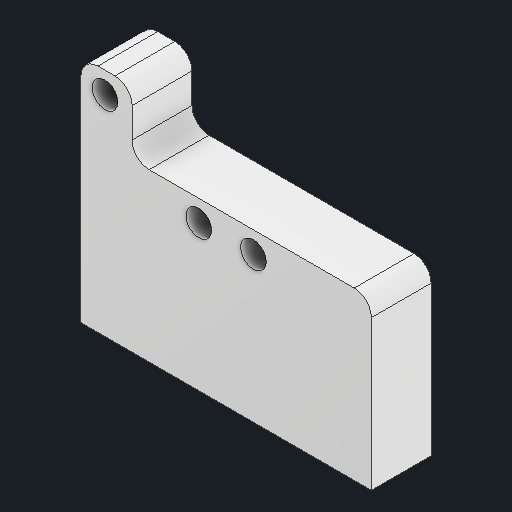
# Autodesk Inventor part: Pixy2Mount
Saved by Autodesk Inventor 2025 (Build 290162000, 162)
## iProperties
Created: 2024-05-22
Part Number: Pixy2Mount
Material: PC/ABS Plastic
Document SubType Name: Modeling
Designer: avsar
Density: 1.1 g/cm^3
Appearance: Smooth - White
Author: avsar
Autodesk Inventor part; units mm, degrees
ref_plane "YZ Plane" through (0, 0, 0) normal (1, 0, 0) x (0, 1, 0)
ref_plane "XZ Plane" through (0, 0, 0) normal (0, 1, 0) x (-1, 0, 0)
ref_plane "XY Plane" through (0, 0, 0) normal (0, 0, 1) x (1, 0, 0)
sketch "Sketch1" plane through (0, 0, 0) normal (0, 1, 0) x (-1, 0, 0)
  circle A0 centre (0, 0) radius 2
  circle A1 centre (12, 0) radius 2
  line L0 (0, 0) -> (0, 2) construction
  circle A2 centre (-12, 0) radius 2
  line L1 (17, 3.5) -> (-17, 3.5)
  line L2 (-17, 3.5) -> (-17, -3.5)
  line L3 (-17, -3.5) -> (17, -3.5)
  line L4 (17, -3.5) -> (17, 3.5)
  line L5 (17, 3.5) -> (-17, -3.5) construction
  line L6 (-17, 3.5) -> (17, -3.5) construction
  dimension "d0" = 4
  dimension "d1" = 4
  dimension "d2" = 12
  dimension "d3" = 34
  dimension "d4" = 7
  constraints: 14 end point, 2 centre point, 2 midpoint, 2 parallel, 1 coincident, 1 horizontal, 1 horizontal alignment, 1 perpendicular, 1 symmetric about line, 1 vertical, 1 vertical alignment, 3 other
  measures "d1" diameter of A1
  measures "d2" distance of point (0, 0) A1.centre
  measures "d3" distance of L3.end L2.end
  measures "d4" distance of L2.end L1.end
extrude "Extrusion1" add sketch "Sketch1" along normal blind 27 contours A0 | A1 | A2 | L4 L3 L2 L1
extrude "Extrusion2" cut sketch "Sketch1" along normal blind 8 contours A0 | A1 | A2
sketch "Sketch2" plane through (-17, 0, 3.5) normal (0, 0, 1) x (1, 0, 0)
  circle A0 centre (20.2, 17) radius 1.5
  circle A1 centre (13.8, 17) radius 1.5
  circle A2 centre (2.825, 24.5) radius 1.5
  line L0 (13.8, 17) -> (20.2, 17) construction
  line L1 (0, 0) -> (34, 0) projected
  line L2 (0, 27) -> (34, 27) construction
  point P0 (17, 0)
  point P1 (17, 17)
  point P2 (17, 0)
  point P3 (17, 27)
  dimension "d9" = 3
  dimension "d10" = 3
  dimension "d11" = 3
  dimension "d12" = 6.4
  dimension "d13" = 10.975
  dimension "d14" = 7.5
  dimension "d15" = 10
  constraints: 3 centre point, 3 midpoint, 2 end point, 1 horizontal, 1 horizontal alignment, 1 vertical alignment
  measures "d9" diameter of A0
  measures "d10" diameter of A1
  measures "d11" diameter of A2
  measures "d12" distance of L0.end L0.start
  measures "d13" horizontal distance of L0.start A2.centre
  measures "d14" vertical distance of A2.centre L0.start
  measures "d15" distance of point (17, 27) point (17, 17)
extrude "Extrusion3" cut sketch "Sketch2" against normal through all
sketch "Sketch3" plane through (-17, 0, 3.5) normal (0, 0, 1) x (1, 0, 0)
  line L0 (34, 27) -> (0, 27) projected
  line L1 (6, 27) -> (6, 19.5)
  line L2 (6, 19.5) -> (34, 19.5)
  line L3 (34, 0) -> (34, 27) projected
  point P0 (17, 0)
  dimension "d18" = 7.5
  dimension "d19" = 28
  constraints: 4 end point, 2 point on line, 1 perpendicular, 1 vertical
  measures "d18" distance of L1.start L1.end
  measures "d19" distance of L1.end L2.end
extrude "Extrusion4" cut sketch "Sketch3" against normal through all
fillet "Fillet1" radius 2 4 edges at (-17, 27, 0) (-11, 27, 0) (-11, 19.5, 0) (17, 19.5, 0)
body "Solid1"
